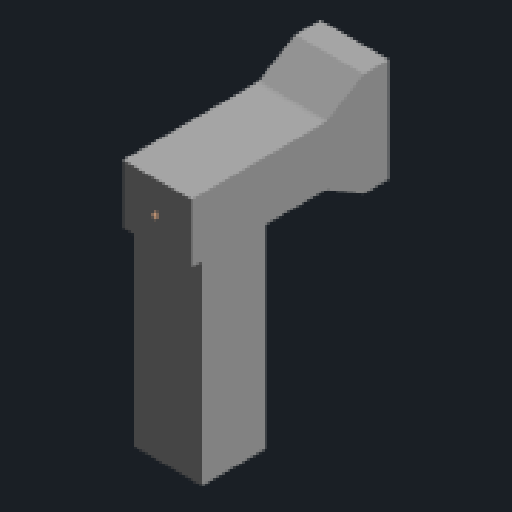
# Autodesk Inventor part: BaseBoundingBox
Saved by Autodesk Inventor 2025.2 (Build 292293000, 293)
## iProperties
Created: 2023-03-25
Part Number: BaseBoundingBox
Material: Generic
Document SubType Name: Modeling
Designer: Val
Density: 1 g/cm^3
Appearance: Default
Author: Val
Autodesk Inventor part; units mm, degrees
ref_plane "YZ Plane" through (0, 0, 0) normal (1, 0, 0) x (0, 1, 0)
ref_plane "XZ Plane" through (0, 0, 0) normal (0, 1, 0) x (-1, 0, 0)
ref_plane "XY Plane" through (0, 0, 0) normal (0, 0, 1) x (1, 0, 0)
sketch "Sketch1" plane through (0, 0, 0) normal (1, 0, 0) x (0, 1, 0)
  line L0 (16, 0) -> (-16, 0)
  line L1 (16, 0) -> (-16, 0) construction
  line L2 (21.5, 0) -> (16, 0)
  line L3 (21.9436, -96.7485) -> (36.9412, -122.057)
  line L4 (21.5, -4) -> (21.5, -95.1299)
  line L5 (21.5, -95.1299) -> (21.9436, -96.7485)
  line L6 (37.5, -124.0962) -> (37.5, -137.065)
  line L7 (36.9412, -122.057) -> (37.5, -123)
  line L8 (37.5, -123) -> (37.5, -124.0962)
  arc A0 (37.5, -124.0962) -> (36.9412, -122.057) centre (33.5, -124.0962) ccw construction
  line L9 (-16, 0) -> (-20.5, 0)
  line L10 (-20.5, 0) -> (-20.5, -95.1299)
  line L11 (-20.5, -95.1299) -> (-20.5, -4) construction
  line L12 (-20.5, -7.5) -> (-159.2, -7.5)
  line L13 (-159.2, -7.5) -> (-159.2, -52.5)
  line L14 (-159.2, -52.5) -> (-20.5, -52.5)
  line L15 (-73.4, -7.5) -> (-107.4, -7.5) construction
  line L16 (-73.4, -52.5) -> (-107.4, -52.5) construction
  line L17 (-159.2, -35.5) -> (-159.2, -24.5) construction
  line L18 (-35.9412, -122.057) -> (-20.9436, -96.7485)
  line L19 (-20.5, -95.1299) -> (-20.9436, -96.7485)
  line L20 (-36.5, -137.065) -> (-36.5, -124.0962)
  arc A1 (-35.9412, -122.057) -> (-36.5, -124.0962) centre (-32.5, -124.0962) ccw construction
  line L21 (-35.9412, -122.057) -> (-36.5, -123)
  line L22 (-36.5, -123) -> (-36.5, -124.0962)
  line L23 (-36.5, -137.065) -> (-36.5, -141)
  line L24 (-36.5, -141) -> (37.5, -141)
  line L25 (37.5, -141) -> (37.5, -137.065)
  line L26 (-36.5, -139.095) -> (-36.5, -141) construction
  line L27 (37.5, -141) -> (37.5, -139.095) construction
  line L28 (-33.325, -141) -> (34.325, -141) construction
  line L29 (21.5, 0) -> (21.5, -4)
  point P0 (0, 0)
  point P1 (0, 0)
  point P2 (21.5, -10)
  point P3 (16, 0)
  point P4 (-20.5, -52.5)
  constraints: 58 end point, 9 collinear, 7 vertical, 4 point on circle, 4 tangent, 3 horizontal, 3 perpendicular, 3 point on line, 2 centre point, 2 coincident, 1 midpoint, 31 other
extrude "Extrusion3" add sketch "Sketch1" along normal mid plane 49
body "Solid2"
